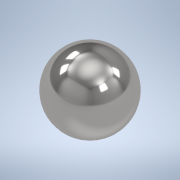
# Autodesk Inventor part: SC8 bearing ball
Saved by Autodesk Inventor 2020.2 (Build 242310000, 310)
## iProperties
Created: 2020-07-09
Part Number: SC8 bearing ball
Material: Ogólny
Document SubType Name: Modeling
Designer: Artur Lenart
Density: 1 g/cm^3
Appearance: Stal — polerowana
Author: Artur Lenart
Autodesk Inventor part; units mm, degrees
ref_plane "YZ Plane" through (0, 0, 0) normal (1, 0, 0) x (0, 1, 0)
ref_plane "XZ Plane" through (0, 0, 0) normal (0, 1, 0) x (-1, 0, 0)
ref_plane "XY Plane" through (0, 0, 0) normal (0, 0, 1) x (1, 0, 0)
sketch "Szkic1" plane through (0, 0, 0) normal (1, 0, 0) x (0, 1, 0)
  circle A0 centre (0, 0) radius 0.75
  line L0 (-0.75, 0) -> (0.75, 0)
  dimension "d0" = 1.5
  constraints: 2 end point, 2 point on circle, 1 centre point, 1 coincident, 1 horizontal
  measures "d0" diameter of A0
revolve "Obrót1" add sketch "Szkic1" angle 360 about axis through (0, -0.75, 0) along (0, 1, 0) picked at (0.1871, 0.1658) contours L0 A0
